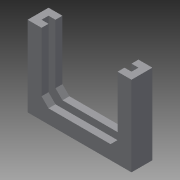
# Autodesk Inventor part: CameraHolder
Saved by Autodesk Inventor 2015 (Build 190159000, 159)
## iProperties
Created: 2015-11-25
Part Number: CameraHolder
Material: Generic
Document SubType Name: Modeling
Designer: Lauszus
Density: 1 g/cm^3
Appearance: Default
Author: Lauszus
Autodesk Inventor part; units mm, degrees
ref_plane "YZ Plane" through (0, 0, 0) normal (1, 0, 0) x (0, 1, 0)
ref_plane "XZ Plane" through (0, 0, 0) normal (0, 1, 0) x (-1, 0, 0)
ref_plane "XY Plane" through (0, 0, 0) normal (0, 0, 1) x (1, 0, 0)
sketch "Sketch1" plane through (0, 0, 0) normal (0, 0, 1) x (1, 0, 0)
  line L0 (-23.4826, 4.2639) -> (2.3174, 4.2639)
  line L1 (2.3174, 4.2639) -> (2.3174, 2.2639)
  line L2 (2.3174, 2.2639) -> (-23.4826, 2.2639)
  line L3 (-23.4826, 2.2639) -> (-23.4826, 4.2639)
  line L4 (-25.4826, 6.2639) -> (4.3174, 6.2639)
  line L5 (4.3174, 6.2639) -> (4.3174, 0.2639)
  line L6 (4.3174, 0.2639) -> (-25.4826, 0.2639)
  line L7 (-25.4826, 0.2639) -> (-25.4826, 6.2639)
  point P0 (0, 0)
  dimension "d0" = 25.8
  dimension "d1" = 2
  dimension "d4" = 2
  dimension "d5" = 2
  dimension "d6" = 2
  dimension "d7" = 2
  constraints: 16 end point, 4 parallel, 2 horizontal, 2 perpendicular
  measures "d0" distance of L0.start L0.end
  measures "d1" distance of L0.end L1.end
  measures "d4" distance between parallel lines of L0 L4
  measures "d5" distance between parallel lines of L3 L7
  measures "d6" distance between parallel lines of L6 L2
  measures "d7" distance between parallel lines of L5 L1
extrude "Extrusion5" add sketch "Sketch1" along normal blind 23 contours L0 L1 L2 L3 | L4 L5 L6 L7
sketch "Sketch4" plane through (0, 0, 23) normal (0, 0, 1) x (1, 0, 0)
  line L0 (-23.4826, 4.2639) -> (2.3174, 4.2639)
  line L1 (2.3174, 4.2639) -> (2.3174, 2.2639)
  line L2 (2.3174, 2.2639) -> (-23.4826, 2.2639)
  line L3 (-23.4826, 2.2639) -> (-23.4826, 4.2639)
  line L4 (-25.4826, 6.2639) -> (-25.4826, 0.2639) projected
  line L5 (4.3174, 6.2639) -> (-25.4826, 6.2639) projected
  line L6 (-25.4826, 0.2639) -> (4.3174, 0.2639) projected
  line L7 (4.3174, 0.2639) -> (4.3174, 6.2639) projected
  point P0 (0, 0)
  dimension "d20" = 2
  dimension "d21" = 2
  dimension "d22" = 2
  dimension "d23" = 2
  constraints: 8 end point, 2 parallel, 1 horizontal, 1 perpendicular
  measures "d20" distance between parallel lines of L4 L3
  measures "d21" distance between parallel lines of L5 L0
  measures "d22" distance between parallel lines of L6 L2
  measures "d23" distance between parallel lines of L7 L1
extrude "Extrusion6" cut sketch "Sketch4" against normal blind 21 contours L0 L1 L2 L3
sketch "Sketch5" plane through (-25.4826, 6.2639, 0) normal (0, 1, 0) x (1, 0, 0)
  line L0 (0, -23) -> (29.8, -23) projected
  line L1 (4, -4) -> (25.8, -4)
  line L2 (25.8, -4) -> (25.8, -23)
  line L3 (25.8, -23) -> (4, -23)
  line L4 (4, -23) -> (4, -4)
  line L5 (0, 0) -> (0, -23) projected
  line L6 (29.8, 0) -> (29.8, -23) projected
  line L7 (0, 0) -> (29.8, 0) projected
  point P0 (25.4826, 0)
  dimension "d26" = 4
  dimension "d27" = 4
  dimension "d28" = 4
  constraints: 8 end point, 2 parallel, 1 horizontal, 1 perpendicular, 1 point on line
  measures "d26" distance between parallel lines of L5 L4
  measures "d27" distance between parallel lines of L6 L2
  measures "d28" distance between parallel lines of L7 L1
extrude "Extrusion7" cut sketch "Sketch5" against normal through all contours L4 L1 L2 L0
chamfer "Chamfer1" distance 2 angle 45 4 edges at (-21.4826, 5.2639, 4) (-21.4826, 1.2639, 4) (0.3174, 5.2639, 4) (0.3174, 1.2639, 4)
body "Solid3"
